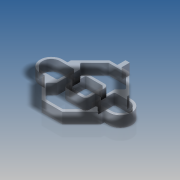
# Autodesk Inventor part: 11026-TransClear
Saved by Autodesk Inventor 2016 SP2 (Build 200236200, 236)
## iProperties
Created: 2015-08-19
Part Number: 11026-TransClear
Material: Polycarbonate
Document SubType Name: Modeling
Designer: D. Kohfeld
Density: 1.2 g/cm^3
Appearance: TransClear
Mass: 1.698 g
Surface Area: 23.7051 cm^2
Volume: 1.415 cm^3
Author: D. Kohfeld
Autodesk Inventor part; units mm, degrees
ref_plane "YZ Plane" through (0, 0, 0) normal (1, 0, 0) x (0, 1, 0)
ref_plane "XZ Plane" through (0, 0, 0) normal (0, 1, 0) x (-1, 0, 0)
ref_plane "XY Plane" through (0, 0, 0) normal (0, 0, 1) x (1, 0, 0)
sketch "Sketch2" plane through (0, 0, 0) normal (0, 1, 0) x (-1, 0, 0)
  line L0 (-3.48, 4.08) -> (3.48, 4.08)
  line L1 (4.08, 3.48) -> (4.08, -3.48)
  line L2 (3.48, -4.08) -> (-3.48, -4.08)
  line L3 (-4.08, -3.48) -> (-4.08, 3.48)
  line L4 (-5.88, 0.6) -> (-7.4, 0.6)
  line L5 (-8, 1.2) -> (-8, 5.36)
  line L6 (-8, 5.36) -> (-10.1957, 7.5557)
  arc A0 (-10.1957, 8.4043) -> (-10.1957, 7.5557) centre (-9.7715, 7.98) ccw
  line L7 (-10.1957, 8.4043) -> (-4, 14.6)
  line L8 (-4, 14.6) -> (4, 14.6)
  line L9 (4, 14.6) -> (10.1957, 8.4043)
  arc A1 (10.1957, 7.5557) -> (10.1957, 8.4043) centre (9.7715, 7.98) ccw
  line L10 (10.1957, 7.5557) -> (8, 5.36)
  line L11 (8, 5.36) -> (8, 1.2)
  line L12 (7.4, 0.6) -> (5.88, 0.6)
  line L13 (-5.88, -0.6) -> (-7.4, -0.6)
  line L14 (-8, -1.2) -> (-8, -5.36)
  line L15 (-8, -5.36) -> (-10.1957, -7.5557)
  arc A2 (-10.1957, -7.5557) -> (-10.1957, -8.4043) centre (-9.7715, -7.98) ccw
  line L16 (-10.1957, -8.4043) -> (-4, -14.6)
  line L17 (-4, -14.6) -> (4, -14.6)
  line L18 (4, -14.6) -> (10.1957, -8.4043)
  arc A3 (10.1957, -8.4043) -> (10.1957, -7.5557) centre (9.7715, -7.98) ccw
  line L19 (10.1957, -7.5557) -> (8, -5.36)
  line L20 (8, -5.36) -> (8, -1.2)
  line L21 (7.4, -0.6) -> (5.88, -0.6)
  line L22 (-9.2, -3.48) -> (-9.2, 3.48)
  line L23 (-9.8, 4.08) -> (-16, 4.08)
  arc A4 (-16, 4.08) -> (-16, -4.08) centre (-16, 0) ccw
  line L24 (-16, -4.08) -> (-9.8, -4.08)
  line L25 (9.2, 3.48) -> (9.2, -3.48)
  line L26 (9.8, -4.08) -> (16, -4.08)
  arc A5 (16, -4.08) -> (16, 4.08) centre (16, 0) ccw
  line L27 (16, 4.08) -> (9.8, 4.08)
  line L28 (13.8, 5.28) -> (13.8, 6.8)
  line L29 (13.8, 6.8) -> (4.8, 15.8)
  line L30 (4.8, 15.8) -> (-4.8, 15.8)
  line L31 (-4.8, 15.8) -> (-13.8, 6.8)
  line L32 (-13.8, 6.8) -> (-13.8, 5.28)
  line L33 (-13.8, 5.28) -> (-16, 5.28)
  arc A6 (-16, 5.28) -> (-16, -5.28) centre (-16, 0) ccw
  line L34 (-16, -5.28) -> (-13.8, -5.28)
  line L35 (-13.8, -5.28) -> (-13.8, -6.4)
  line L36 (-13.8, -6.4) -> (-4.4, -15.8)
  line L37 (-4.4, -15.8) -> (-0.8, -15.8)
  line L38 (-0.8, -15.8) -> (-0.8, -19.6)
  line L39 (-0.8, -19.6) -> (1.2, -19.6)
  line L40 (1.2, -19.6) -> (1.2, -15.8)
  line L41 (1.2, -15.8) -> (4.8, -15.8)
  line L42 (4.8, -15.8) -> (13.8, -6.8)
  line L43 (13.8, -6.8) -> (13.8, -5.28)
  line L44 (13.8, -5.28) -> (16, -5.28)
  arc A7 (16, -5.28) -> (16, 5.28) centre (16, 0) ccw
  line L45 (16, 5.28) -> (13.8, 5.28)
  arc A8 (-3.48, 4.08) -> (-4.08, 3.48) centre (-3.48, 3.48) ccw
  arc A9 (4.08, 3.48) -> (3.48, 4.08) centre (3.48, 3.48) ccw
  arc A10 (-4.08, -3.48) -> (-3.48, -4.08) centre (-3.48, -3.48) ccw
  arc A11 (3.48, -4.08) -> (4.08, -3.48) centre (3.48, -3.48) ccw
  arc A12 (-8, 1.2) -> (-7.4, 0.6) centre (-7.4, 1.2) ccw
  arc A13 (-5.88, 0.6) -> (-5.28, 1.2) centre (-5.88, 1.2) ccw
  arc A14 (-5.28, -1.2) -> (-5.88, -0.6) centre (-5.88, -1.2) ccw
  arc A15 (-7.4, -0.6) -> (-8, -1.2) centre (-7.4, -1.2) ccw
  arc A16 (5.28, 1.2) -> (5.88, 0.6) centre (5.88, 1.2) ccw
  arc A17 (7.4, 0.6) -> (8, 1.2) centre (7.4, 1.2) ccw
  arc A18 (5.88, -0.6) -> (5.28, -1.2) centre (5.88, -1.2) ccw
  arc A19 (8, -1.2) -> (7.4, -0.6) centre (7.4, -1.2) ccw
  line L46 (-5.28, 1.2) -> (-5.28, 3.48)
  arc A20 (-3.48, 5.28) -> (-5.28, 3.48) centre (-3.48, 3.48) ccw
  line L47 (-3.48, 5.28) -> (3.48, 5.28)
  arc A21 (5.28, 3.48) -> (3.48, 5.28) centre (3.48, 3.48) ccw
  line L48 (5.28, 3.48) -> (5.28, 1.2)
  line L49 (5.28, -1.2) -> (5.28, -3.48)
  arc A22 (3.48, -5.28) -> (5.28, -3.48) centre (3.48, -3.48) ccw
  line L50 (3.48, -5.28) -> (-3.48, -5.28)
  arc A23 (-5.28, -3.48) -> (-3.48, -5.28) centre (-3.48, -3.48) ccw
  line L51 (-5.28, -3.48) -> (-5.28, -1.2)
  arc A24 (-9.2, 3.48) -> (-9.8, 4.08) centre (-9.8, 3.48) ccw
  arc A25 (-9.8, -4.08) -> (-9.2, -3.48) centre (-9.8, -3.48) ccw
  arc A26 (9.8, 4.08) -> (9.2, 3.48) centre (9.8, 3.48) ccw
  arc A27 (9.2, -3.48) -> (9.8, -4.08) centre (9.8, -3.48) ccw
  point P0 (0, 0)
  point P1 (-4.08, 0)
  point P2 (0, 4.08)
  point P3 (0, 15.8)
  point P4 (0, 14.6)
  dimension "d0" = 0.6
  dimension "d1" = 0.6
  dimension "d2" = 0.6
  dimension "d3" = 8.16
  dimension "d4" = 1.2
  dimension "d5" = 1.2
  dimension "d6" = 2.72
  dimension "d7" = 10.72
  dimension "d8" = 1.2
  dimension "d9" = 1.2
  dimension "d10" = 6.8
  dimension "d11" = 10.56
  dimension "d12" = 27.6
  dimension "d13" = 13.2
  dimension "d14" = 31.6
  dimension "d15" = 15.8
  dimension "d16" = 9.6
  dimension "d17" = 1.2
  dimension "d18" = 8
  dimension "d19" = 2
  dimension "d20" = 3.8
  constraints: 104 end point, 56 point on circle, 51 tangent, 28 centre point, 21 horizontal, 18 equal length, 18 equal radius, 16 vertical, 11 collinear, 7 parallel, 7 perpendicular, 5 concentric, 4 midpoint, 3 vertical alignment, 1 coincident, 1 horizontal alignment
  measures "d0" radius of A8
  measures "d1" radius of A12
  measures "d2" radius of A24
  measures "d3" distance between parallel lines of L2 L0
  measures "d4" distance between parallel lines of L47 L0
  measures "d5" distance between parallel lines of L4 L13
  measures "d6" distance between parallel lines of L46 L5
  measures "d7" distance of L14.end L5.end
  measures "d8" distance between parallel lines of L22 L5
  measures "d9" distance between parallel lines of L25 L11
  measures "d10" distance from line of A4.centre L22
  measures "d11" diameter of A6
  measures "d12" distance between parallel lines of L28 L32
  measures "d13" distance of L35.end L31.end
  measures "d14" distance between parallel lines of L37 L30
  measures "d15" distance from line of L30 A4.centre
  measures "d16" distance of L29.end L30.end
  measures "d17" distance between parallel lines of L30 L8
  measures "d18" distance of L7.end L8.end
  measures "d19" distance of L38.end L39.end
  measures "d20" distance between parallel lines of L39 L37
extrude "Extrusion1" add sketch "Sketch2" along normal mid plane 5.2
fillet "Fillet1" radius 0.1 174 edges at (-14.9, 2.6, 5.28) (-14.9, 2.6, -5.28) (-21.28, 2.6, 0) (-13.8, 2.6, 6.04) (-9.3, 2.6, 11.3) (0, 2.6, 15.8) (9.3, 2.6, 11.3) (13.8, 2.6, 6.04) (21.28, 2.6, 0) (14.9, 2.6, -5.28) (14.9, 2.6, 5.28) (13.8, 2.6, -5.84) (9.1, 2.6, -11.1) (2.6, 2.6, -15.8) (0.8, 2.6, -17.7) (-0.2, 2.6, -19.6) (-1.2, 2.6, -17.7) (-3, 2.6, -15.8) (-9.3, 2.6, -11.3) (-13.8, 2.6, -6.04) (-14.9, -2.6, -5.28) (-14.9, -2.6, 5.28) (-21.28, -2.6, 0) (-13.8, -2.6, 6.04) (0, -2.6, 15.8) (9.3, -2.6, 11.3) (-9.3, -2.6, 11.3) (13.8, -2.6, 6.04) (21.28, -2.6, 0) (14.9, -2.6, -5.28) (14.9, -2.6, 5.28) (13.8, -2.6, -5.84) (13.8, 0, -6.4) (9.1, -2.6, -11.1) (2.6, -2.6, -15.8) (0.8, -2.6, -17.7) (-0.2, -2.6, -19.6) (-1.2, -2.6, -17.7) (-3, -2.6, -15.8) (-9.3, -2.6, -11.3) (-13.8, -2.6, -6.04) (-4.8, 0, 15.8) (4.8, 0, 15.8) (13.8, 0, 6.8) (4.4, 0, -15.8) (0.8, 0, -19.6) (-1.2, 0, -19.6) (-4.8, 0, -15.8) (-13.8, 0, -6.8) (-13.8, 0, 6.8) (-12.9, 2.6, -4.08) (-9.3757, 2.6, -3.9043) (-9.2, 2.6, 0) (-9.3757, 2.6, 3.9043) (-12.9, 2.6, 4.08) (-20.08, 2.6, 0) (-12.9, -2.6, 4.08) (-9.3757, -2.6, 3.9043) (-9.2, -2.6, 0) (-9.3757, -2.6, -3.9043) (-12.9, -2.6, -4.08) (-20.08, -2.6, 0) (9.3757, 2.6, -3.9043) (12.9, 2.6, -4.08) (20.08, 2.6, 0) (12.9, 2.6, 4.08) (9.3757, 2.6, 3.9043) (9.2, 2.6, 0) (9.3757, -2.6, 3.9043) (12.9, -2.6, 4.08) (20.08, -2.6, 0) (12.9, -2.6, -4.08) (9.3757, -2.6, -3.9043) (9.2, -2.6, 0) (3.9043, 2.6, -3.9043) (4.08, 2.6, 0) (3.9043, 2.6, 3.9043) (0, 2.6, 4.08) (-3.9043, 2.6, 3.9043) (-4.08, 2.6, 0) (-3.9043, 2.6, -3.9043) (0, 2.6, -4.08) (-3.9043, -2.6, -3.9043) (-4.08, -2.6, 0) (-3.9043, -2.6, 3.9043) (0, -2.6, 4.08) (3.9043, -2.6, 3.9043) (4.08, -2.6, 0) (3.9043, -2.6, -3.9043) (0, -2.6, -4.08) (5.4557, 2.6, 0.7757) (6.64, 2.6, 0.6) (7.8243, 2.6, 0.7757) (8, 2.6, 3.28) (4.7528, 2.6, 4.7528) (0, 2.6, 5.28) (-4.7528, 2.6, 4.7528) (-5.28, 2.6, 2.34) (-5.4557, 2.6, 0.7757) (-6.64, 2.6, 0.6) (-7.8243, 2.6, 0.7757) (-8, 2.6, 3.28) (5.28, 2.6, 2.34) (0, 2.6, -5.28) (-4.7528, 2.6, -4.7528) (-5.28, 2.6, -2.34) (-5.4557, 2.6, -0.7757) (-6.64, 2.6, -0.6) (-7.8243, 2.6, -0.7757) (-8, 2.6, -3.28) (5.28, 2.6, -2.34) (5.4557, 2.6, -0.7757) (6.64, 2.6, -0.6) (7.8243, 2.6, -0.7757) (8, 2.6, -3.28) (4.7528, 2.6, -4.7528) (-4.7528, -2.6, 4.7528) (-5.28, -2.6, 2.34) (-5.4557, -2.6, 0.7757) (-6.64, -2.6, 0.6) (-7.8243, -2.6, 0.7757) (-8, -2.6, 3.28) (4.7528, -2.6, 4.7528) (5.28, -2.6, 2.34) (5.4557, -2.6, 0.7757) (6.64, -2.6, 0.6) (7.8243, -2.6, 0.7757) (8, -2.6, 3.28) (0, -2.6, 5.28) (0, -2.6, -5.28) (4.7528, -2.6, -4.7528) (5.28, -2.6, -2.34) (5.4557, -2.6, -0.7757) (6.64, -2.6, -0.6) (7.8243, -2.6, -0.7757) (8, -2.6, -3.28) (-5.28, -2.6, -2.34) (-5.4557, -2.6, -0.7757) (-6.64, -2.6, -0.6) (-7.8243, -2.6, -0.7757) (-8, -2.6, -3.28) (-4.7528, -2.6, -4.7528) (8, 0, 5.36) (8, 0, -5.36) (-8, 0, -5.36) (-8, 0, 5.36) (-10.3715, 2.6, 7.98) (-7.0979, 2.6, 11.5021) (-9.0979, 2.6, 6.4579) (-10.3715, -2.6, 7.98) (-7.0979, -2.6, 11.5021) (-9.0979, -2.6, 6.4579) (0, 2.6, 14.6) (0, -2.6, 14.6) (10.3715, 2.6, 7.98) (9.0979, 2.6, 6.4579) (7.0979, 2.6, 11.5021) (10.3715, -2.6, 7.98) (9.0979, -2.6, 6.4579) (7.0979, -2.6, 11.5021) (10.3715, 2.6, -7.98) (7.0979, 2.6, -11.5021) (9.0979, 2.6, -6.4579) (10.3715, -2.6, -7.98) (7.0979, -2.6, -11.5021) (9.0979, -2.6, -6.4579) (0, -2.6, -14.6) (0, 2.6, -14.6) (-10.3715, -2.6, -7.98) (-9.0979, -2.6, -6.4579) (-7.0979, -2.6, -11.5021) (-10.3715, 2.6, -7.98) (-9.0979, 2.6, -6.4579) (-7.0979, 2.6, -11.5021)
equation "\"d9\" = d8"
equation "\"d18\" = lu"
equation "\"lu\" = 8"
body "Solid1"
